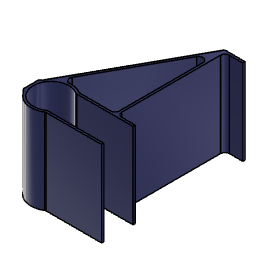
Endstop Clip v3 v2 (Autodesk Fusion 360 design; units mm, degrees)
Autodesk Fusion 360 part; units mm, degrees
sketch "Sketch1" plane through (0, 0, 0) normal (0, 0, 1) x (1, 0, 0)
  line L0 (0, 0) -> (-25.0251, 0)
  line L1 (0, 15) -> (-25.0251, 15)
  arc A0 (-25.0251, 15) -> (-25.0251, 0) centre (-30, 7.5) ccw
  line L2 (0, 1) -> (-25.3363, 1)
  arc A1 (-25.3363, 14) -> (-25.3363, 1) centre (-30, 7.5) ccw
  line L3 (0, 14) -> (-25.3363, 14)
  line L4 (0, 15) -> (-8, 15)
  line L5 (-8, 15) -> (-8, 63)
  line L6 (-8, 63) -> (0, 63)
  line L7 (0, 14) -> (-9, 14)
  line L8 (-9, 64) -> (0, 64)
  line L9 (-9, 64) -> (-37.8734, 11.86)
  line L10 (-39, 7.5) -> (-39, 11)
  line L11 (-39, 7.5) -> (-39, 4)
  line L12 (-39, 7.5) -> (-36.2777, 7.5)
  line L13 (-37.8734, 11.86) -> (-39, 11)
  line L14 (-37.8734, 3.14) -> (-39, 4)
  line L15 (-9, 61.9358) -> (-35.0011, 14.9826)
  line L16 (-9, 15) -> (-9, 61.9358)
  line L17 (0, 15) -> (0, 14)
  line L18 (0, 1) -> (0, 0)
  line L19 (0, 64) -> (0, 63)
  dimension "d2" = 15
  dimension "d4" = 18
  dimension "d5" = 1
  dimension "d6" = 8
  dimension "d7" = 48
  dimension "d8" = 8
  dimension "d10" = 3.5
  dimension "d11" = 3.5
  constraint coincident L0.start L18.end
  constraint horizontal L0
  constraint parallel L1 L4
  constraint perpendicular L1 L5
  constraint perpendicular L5 L6
  constraint parallel L4 L7
  constraint parallel L6 L8
  constraint coincident A0 L9.end
  constraint tangent A0 L9
  constraint midpoint A0 L10.start
  constraint vertical L10
  constraint parallel L10 L11
  constraint perpendicular L11 L12
  constraint symmetric L9.end L12 L14.start
  constraint symmetric L10.end L12 L11.end
  constraint parallel L9 L15
  constraint coincident A0 L15.end
  constraint coincident L1 L16.start
  constraint perpendicular L8 L16
  constraint perpendicular L7 L17
  constraint perpendicular L0 L18
  constraint perpendicular L6 L19
  measures "d2" distance of L0.start L1.start
  measures "d4" diameter of A0
  measures "d6" distance of L1.start L4.end
  measures "d7" distance of L4.end L5.end
  measures "d8" distance of L5.end L6.end
  measures "d10" distance of L10.start L10.end
  measures "d11" distance of L10.start L11.end
extrude "Extrude1" add sketch "Sketch1" along normal blind 38 contours L0 A0 L2 A1 L12 L18 | A0 L11 L14 | A0 L10 L13 | L1 A0 A1 L3 L4 L7 L12 L17 | L1 A0 L5 L6 L8 L9 L15 L16 L19 makes body 1
fillet "Fillet1" radius 2 2 edges at (-9, 15, 19) (-8, 15, 19) on bodies 1
fillet "Fillet2" radius 2 1 edges at (-9, 61.9358, 19) on bodies 1
fillet "Fillet2" radius 2 1 edges at (-35.0011, 14.9826, 19) on bodies 1
fillet "Fillet3" radius 2 1 edges at (-8, 63, 19) on bodies 1
fillet "Fillet3" radius 1 2 edges at (-25.0251, 0, 19) (-25.0251, 15, 19) on bodies 1
fillet "Fillet3" radius 1 2 edges at (-25.3363, 14, 19) (-25.3363, 1, 19) on bodies 1
fillet "Fillet4" radius 1 4 edges at (-37.8734, 11.86, 19) (-39, 11, 19) (-39, 4, 19) (-37.8734, 3.14, 19) on bodies 1
extrude "Extrude2" add 1 faces at (-18.5906, 46.6811, 12.6667) along direction (-0.874821, 0.484447, 0) blind 0.1 separate body on bodies 1 makes body 2
